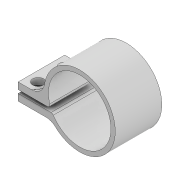
# Autodesk Inventor part: Halterung_Akku_210403
Saved by Autodesk Inventor 2020 (Build 240168000, 168)
## iProperties
Created: 2020-11-08
Part Number: Halterung_Akku_210403
Material: Generisch
Document SubType Name: Modeling
Designer: uhlma
Density: 1 g/cm^3
Appearance: Vorgabe
Author: uhlma
Autodesk Inventor part; units mm, degrees
ref_plane "YZ Plane" through (0, 0, 0) normal (1, 0, 0) x (0, 1, 0)
ref_plane "XZ Plane" through (0, 0, 0) normal (0, 1, 0) x (-1, 0, 0)
ref_plane "XY Plane" through (0, 0, 0) normal (0, 0, 1) x (1, 0, 0)
sketch "Skizze1" plane through (0, 0, 0) normal (0, 0, 1) x (1, 0, 0)
  arc A0 (-8.1406, -4.7) -> (-8.6412, -3.7) centre (0, 0) ccw
  line L0 (-18.5, -6.7) -> (-8.3427, -6.7)
  line L1 (-18.5, -6.7) -> (-18.5, -4.7)
  line L2 (-18.5, -4.7) -> (-8.1406, -4.7)
  line L3 (-18.5, -1.7) -> (-18.5, -3.7)
  line L4 (-18.5, -3.7) -> (-8.6412, -3.7)
  line L5 (-18.5, -1.7) -> (-14.519, -1.7)
  arc A1 (-8.3427, -6.7) -> (-10.5682, 1.6741) centre (0, 0) ccw
  arc A2 (-14.519, -1.7) -> (-10.5682, 1.6741) centre (-14.519, 2.3) ccw
  point P0 (-10.5641, -1.7)
  dimension "d0" = 18.8
  dimension "d2" = 2
  dimension "d4" = 1
  dimension "d5" = 18.5
  dimension "d6" = 4
  dimension "d7" = 1.3
  dimension "d19" = 10.1573
  dimension "d26" = 4
  constraints: 12 end point, 7 point on circle, 3 centre point, 3 point on line, 2 coincident, 2 perpendicular, 2 tangent, 1 collinear, 1 horizontal, 1 parallel, 1 vertical
  measures "d0" diameter of A0
  measures "d2" distance of L0.start L1.end
  measures "d4" distance between parallel lines of L4 L2
  measures "d5" distance from line of A1.centre L1
  measures "d6" distance edge to line of A1 L0
  measures "d7" radial gap between concentric circles of A1 A0
  measures "d19" distance of L0.end L0.start
  measures "d26" radius of A2
extrude "Extrusion1" add sketch "Skizze1" along normal mid plane 14
sketch "Skizze2" plane through (-18.5, -1.7, 7) normal (0, 1, 0) x (1, 0, 0)
  circle A0 centre (3, 11) radius 1.65
  line L0 (0, 14) -> (3.981, 14) projected
  line L1 (0, 14) -> (0, 0) projected
  line L2 (0, 14) -> (0, 0) construction
  line L3 (0, 7) -> (7.2294, 7) construction
  circle A1 centre (3, 3) radius 1.65
  circle A2 centre (3, 11) radius 3
  circle A3 centre (3, 3) radius 3
  point P0 (18.5, 7)
  point P1 (9.0709, 16)
  point P2 (0, 3)
  point P3 (0, 0.6676)
  point P4 (0.6676, 16)
  point P5 (0, 11)
  point P6 (0, 10.6676)
  point P7 (3, 14)
  dimension "d10" = 3
  dimension "d11" = 3
  dimension "d12" = 3.3
  dimension "d20" = 6
  constraints: 4 centre point, 2 coincident, 2 end point, 1 equal radius, 1 horizontal, 1 midpoint, 1 symmetric about line, 2 other
  measures "d11" distance from line of A0.centre L1
  measures "d12" diameter of A0
  measures "d20" diameter of A2
extrude "Extrusion2" cut sketch "Skizze2" against normal through all both and the other way through all contours A0 | A1
fillet "Rundung2" radius 4 1 edges at (-8.3427, -6.7, 0)
fillet "Rundung3" radius 0.8 2 edges at (-8.6412, -3.7, 0) (-8.1406, -4.7, 0)
extrude "Extrusion4" cut sketch "Skizze2" along normal blind 10 contours A3 | A2
